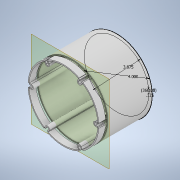
# Autodesk Inventor part: Main Iris box
Saved by Autodesk Inventor 2021 (Build 250183000, 183)
## iProperties
Created: 2020-07-09
Part Number: Main Iris box
Material: Generic
Document SubType Name: Modeling
Designer: saipr
Density: 1 g/cm^3
Appearance: Default
Author: saipr
Autodesk Inventor part; units mm, degrees
ref_plane "YZ Plane" through (0, 0, 0) normal (1, 0, 0) x (0, 1, 0)
ref_plane "XZ Plane" through (0, 0, 0) normal (0, 1, 0) x (-1, 0, 0)
ref_plane "XY Plane" through (0, 0, 0) normal (0, 0, 1) x (1, 0, 0)
sketch "Sketch1" plane through (0, 0, 0) normal (0, 0, 1) x (1, 0, 0)
  circle A0 centre (0, 0) radius 50.8
  circle A1 centre (0, 0) radius 49.2125
  line L0 (49.2125, 0) -> (46.0375, 0)
  arc A2 (46.0375, 3.175) -> (46.0375, -3.175) centre (46.0375, 0) ccw
  arc A3 (46.0375, 1.5875) -> (46.0375, -1.5875) centre (46.0375, 0) ccw
  line L1 (46.0375, -3.175) -> (50.7007, -3.175)
  line L2 (46.0375, 3.175) -> (50.7007, 3.175)
  line L3 (46.0375, 1.5875) -> (49.1869, 1.5875)
  line L4 (46.0375, -1.5875) -> (49.1869, -1.5875)
  line L5 (20.2691, 41.4571) -> (22.6007, 45.4956)
  arc A4 (20.2691, 41.4571) -> (25.7684, 38.2821) centre (23.0188, 39.8696) ccw
  line L6 (21.6439, 40.6634) -> (23.2186, 43.3908)
  arc A5 (21.6439, 40.6634) -> (24.3936, 39.0759) centre (23.0188, 39.8696) ccw
  line L7 (25.7684, 38.2821) -> (28.1, 42.3206)
  line L8 (-25.7684, 38.2821) -> (-28.1, 42.3206)
  arc A6 (-25.7684, 38.2821) -> (-20.2691, 41.4571) centre (-23.0187, 39.8696) ccw
  line L9 (-24.3936, 39.0759) -> (-25.9683, 41.8033)
  arc A7 (-24.3936, 39.0759) -> (-21.6439, 40.6634) centre (-23.0187, 39.8696) ccw
  line L10 (-20.2691, 41.4571) -> (-22.6007, 45.4956)
  line L11 (-46.0375, -3.175) -> (-50.7007, -3.175)
  arc A8 (-46.0375, -3.175) -> (-46.0375, 3.175) centre (-46.0375, 0) ccw
  line L12 (-46.0375, -1.5875) -> (-49.1869, -1.5875)
  arc A9 (-46.0375, -1.5875) -> (-46.0375, 1.5875) centre (-46.0375, 0) ccw
  line L13 (-46.0375, 3.175) -> (-50.7007, 3.175)
  line L14 (-20.2691, -41.4571) -> (-22.6007, -45.4956)
  arc A10 (-20.2691, -41.4571) -> (-25.7684, -38.2821) centre (-23.0188, -39.8696) ccw
  line L15 (-21.6439, -40.6634) -> (-23.2186, -43.3908)
  arc A11 (-21.6439, -40.6634) -> (-24.3936, -39.0759) centre (-23.0188, -39.8696) ccw
  line L16 (-25.7684, -38.2821) -> (-28.1, -42.3206)
  line L17 (25.7684, -38.2821) -> (28.1, -42.3206)
  arc A12 (25.7684, -38.2821) -> (20.2691, -41.4571) centre (23.0187, -39.8696) ccw
  line L18 (24.3936, -39.0759) -> (25.9683, -41.8033)
  arc A13 (24.3936, -39.0759) -> (21.6439, -40.6634) centre (23.0187, -39.8696) ccw
  line L19 (20.2691, -41.4571) -> (22.6007, -45.4956)
  line L20 (-46.0375, 1.5875) -> (-49.1869, 1.5875)
  line L21 (-21.6439, 40.6634) -> (-23.2186, 43.3908)
  line L22 (24.3936, 39.0759) -> (25.9683, 41.8033)
  line L23 (21.6439, -40.6634) -> (23.0583, -43.4763)
  line L24 (-24.3936, -39.0759) -> (-25.9683, -41.8033)
  point P0 (49.11, -3.175)
  point P1 (49.11, 3.175)
  point P2 (-49.11, 3.175)
  point P3 (-27.3046, 40.943)
  point P4 (-21.8054, 44.118)
  point P5 (21.8054, 44.118)
  point P6 (-27.3046, -40.943)
  point P7 (-49.11, -3.175)
  point P8 (21.8054, -44.118)
  point P9 (-21.8054, -44.118)
  point P10 (27.3046, -40.943)
  point P11 (27.3046, 40.943)
  dimension "d1" = 98.425
  dimension "d0" = 101.6
  dimension "d6" = 3.175
  dimension "d7" = 3.175
  dimension "d24" = 360
  constraints: 50 end point, 26 point on circle, 13 centre point, 9 coincident, 4 horizontal, 3 parallel, 95 other
  measures "d0" diameter of A0
  measures "d6" distance of L0.start L0.end
  measures "d7" diameter of A3
extrude "Extrusion1" add sketch "Sketch1" along normal blind 6.35 contours L2 A2 L1 A1 L17 A12 L19 L14 A10 L16 L11 A8 L13 L8 A6 L10 L5 A4 L7 | A1 L3 A3 L4 L1 A2 L2 | L7 A4 L5 A1 L6 A5 L22 | A1 L4 A3 L3 | A1 L18 A13 L23 L19 A12 L17 | L22 A5 L6 A1 | A1 L23 A13 L18 | L10 A6 L8 A1 L9 A7 L21 | A1 L15 A11 L24 L16 A10 L14 | L21 A7 L9 A1 | A1 L24 A11 L15 | L13 A8 L11 A1 L12 A9 L20 | L20 A9 L12 A1
extrude "Extrusion6" add sketch "Sketch1" along normal blind 76.2 contours L2 A1 L7 A0 | A0 L17 A1 L1 | L5 A1 L10 A0 | A0 L14 A1 L19 | L8 A1 L13 A0 | A0 L11 A1 L16
extrude "Extrusion7" add sketch "Sketch1" along normal blind 63.5 contours A0 L1 A1 L2 | L7 A1 L5 A0 | A0 L19 A1 L17 | L10 A1 L8 A0 | A0 L16 A1 L14 | L13 A1 L11 A0
extrude "Extrusion8" add sketch "Sketch1" along normal blind 76.2 contours A1 L3 A3 L4 L1 A2 L2 | L7 A4 L5 A1 L6 A5 L22 | A1 L18 A13 L23 L19 A12 L17 | L10 A6 L8 A1 L9 A7 L21 | A1 L15 A11 L24 L16 A10 L14 | L13 A8 L11 A1 L12 A9 L20
ref_plane "Work Plane1" through (0, 0, 66.675) normal (0, 0, -1) x (-1, 0, 0)
sketch "Sketch2" plane through (0, 0, 66.675) normal (0, 0, -1) x (-1, 0, 0)
  circle A0 centre (0, 0) radius 50.8
  circle A1 centre (0, 0) radius 49.2125
  dimension "d33" = 101.6
  dimension "d34" = 98.425
  constraints: 2 centre point, 2 coincident
  measures "d33" diameter of A0
  measures "d34" diameter of A1
extrude "Extrusion9" cut sketch "Sketch2" along normal blind 3.175
body "Solid1"
